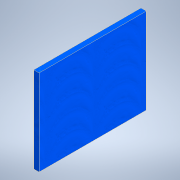
# Autodesk Inventor part: Aurdino
Saved by Autodesk Inventor 2022.2 (Build 262287000, 287)
## iProperties
Created: 2022-02-23
Part Number: Aurdino
Material: PVC-Piping
Document SubType Name: Modeling
Designer: PRASHANTH
Density: 1.4 g/cm^3
Appearance: Weld - Brass
Author: PRASHANTH
Autodesk Inventor part; units mm, degrees
ref_plane "YZ Plane" through (0, 0, 0) normal (1, 0, 0) x (0, 1, 0)
ref_plane "XZ Plane" through (0, 0, 0) normal (0, 1, 0) x (-1, 0, 0)
ref_plane "XY Plane" through (0, 0, 0) normal (0, 0, 1) x (1, 0, 0)
sketch "Sketch1" plane through (0, 0, 0) normal (1, 0, 0) x (0, 1, 0)
  line L0 (-40, 50) -> (40, 50)
  line L1 (40, 50) -> (40, -50)
  line L2 (40, -50) -> (-40, -50)
  line L3 (-40, -50) -> (-40, 50)
  line L4 (-40, 50) -> (40, -50) construction
  line L5 (40, 50) -> (-40, -50) construction
  point P0 (0, 0)
  dimension "d0" = 80
  dimension "d1" = 100
  constraints: 12 end point, 2 midpoint, 2 parallel, 1 horizontal, 1 perpendicular
  measures "d0" distance of L1.end L2.end
  measures "d1" distance of L0.end L1.end
extrude "Extrusion1" add sketch "Sketch1" along normal blind 5
body "Solid1"
